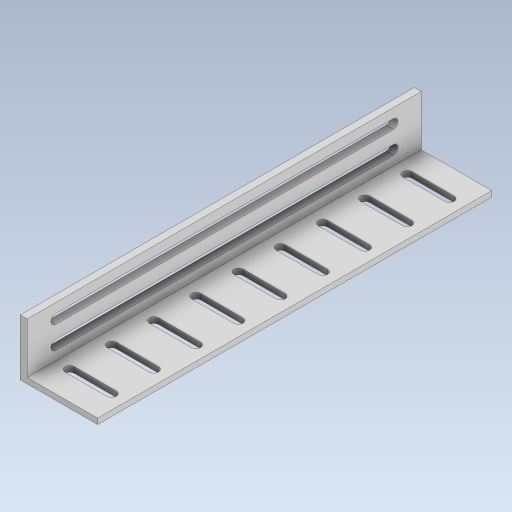
# Autodesk Inventor part: Alas Conveyor
Saved by Autodesk Inventor 2023.5 (Build 275446000, 446)
## iProperties
Created: 2025-10-12
Part Number: Alas Conveyor
Material: Generic
Document SubType Name: Modeling
Designer: Guntur
Density: 1 g/cm^3
Appearance: Default
Author: Guntur
Autodesk Inventor part; units mm, degrees
ref_plane "YZ Plane" through (0, 0, 0) normal (1, 0, 0) x (0, 1, 0)
ref_plane "XZ Plane" through (0, 0, 0) normal (0, 1, 0) x (-1, 0, 0)
ref_plane "XY Plane" through (0, 0, 0) normal (0, 0, 1) x (1, 0, 0)
sketch "Sketch1" plane through (0, 0, 0) normal (0, 1, 0) x (-1, 0, 0)
  line L0 (0, 0) -> (-27.5, 0)
  line L1 (-27.5, 0) -> (-27.5, -140)
  line L2 (-27.5, -140) -> (0, -140)
  line L3 (0, -140) -> (0, 0)
  line L4 (0, 0) -> (-2.5, 0)
  line L5 (-2.5, 0) -> (-2.5, -140)
  line L6 (-2.5, -140) -> (0, -140)
  line L7 (0, -140) -> (0, 0)
  arc A0 (-7.5, -11.65) -> (-7.5, -8.35) centre (-7.5, -10) ccw
  arc A1 (-22.5, -8.35) -> (-22.5, -11.65) centre (-22.5, -10) ccw
  line L8 (-7.5, -11.65) -> (-22.5, -11.65)
  line L9 (-22.5, -8.35) -> (-7.5, -8.35)
  arc A2 (-7.5, -26.65) -> (-7.5, -23.35) centre (-7.5, -25) ccw
  line L10 (-22.5, -23.35) -> (-7.5, -23.35)
  line L11 (-7.5, -26.65) -> (-22.5, -26.65)
  arc A3 (-22.5, -23.35) -> (-22.5, -26.65) centre (-22.5, -25) ccw
  arc A4 (-7.5, -41.65) -> (-7.5, -38.35) centre (-7.5, -40) ccw
  line L12 (-22.5, -38.35) -> (-7.5, -38.35)
  line L13 (-7.5, -41.65) -> (-22.5, -41.65)
  arc A5 (-22.5, -38.35) -> (-22.5, -41.65) centre (-22.5, -40) ccw
  arc A6 (-7.5, -56.65) -> (-7.5, -53.35) centre (-7.5, -55) ccw
  line L14 (-22.5, -53.35) -> (-7.5, -53.35)
  line L15 (-7.5, -56.65) -> (-22.5, -56.65)
  arc A7 (-22.5, -53.35) -> (-22.5, -56.65) centre (-22.5, -55) ccw
  arc A8 (-7.5, -71.65) -> (-7.5, -68.35) centre (-7.5, -70) ccw
  line L16 (-22.5, -68.35) -> (-7.5, -68.35)
  line L17 (-7.5, -71.65) -> (-22.5, -71.65)
  arc A9 (-22.5, -68.35) -> (-22.5, -71.65) centre (-22.5, -70) ccw
  arc A10 (-7.5, -86.65) -> (-7.5, -83.35) centre (-7.5, -85) ccw
  line L18 (-22.5, -83.35) -> (-7.5, -83.35)
  line L19 (-7.5, -86.65) -> (-22.5, -86.65)
  arc A11 (-22.5, -83.35) -> (-22.5, -86.65) centre (-22.5, -85) ccw
  arc A12 (-7.5, -101.65) -> (-7.5, -98.35) centre (-7.5, -100) ccw
  line L20 (-22.5, -98.35) -> (-7.5, -98.35)
  line L21 (-7.5, -101.65) -> (-22.5, -101.65)
  arc A13 (-22.5, -98.35) -> (-22.5, -101.65) centre (-22.5, -100) ccw
  arc A14 (-7.5, -116.65) -> (-7.5, -113.35) centre (-7.5, -115) ccw
  line L22 (-22.5, -113.35) -> (-7.5, -113.35)
  line L23 (-7.5, -116.65) -> (-22.5, -116.65)
  arc A15 (-22.5, -113.35) -> (-22.5, -116.65) centre (-22.5, -115) ccw
  arc A16 (-7.5, -131.65) -> (-7.5, -128.35) centre (-7.5, -130) ccw
  line L24 (-22.5, -128.35) -> (-7.5, -128.35)
  line L25 (-7.5, -131.65) -> (-22.5, -131.65)
  arc A17 (-22.5, -128.35) -> (-22.5, -131.65) centre (-22.5, -130) ccw
  dimension "d0" = 27.5
  dimension "d1" = 140
  dimension "d2" = 2.5
  dimension "d21" = 3.3
  dimension "d22" = 10
  dimension "d23" = 5
  dimension "d24" = 3.3
  dimension "d25" = 5
  dimension "d28" = 15
  constraints: 52 end point, 36 point on circle, 18 centre point, 5 parallel, 3 horizontal, 2 perpendicular, 1 point on line, 1 vertical, 80 other
  measures "d0" distance of L2.end L1.end
  measures "d1" distance of L1.end L0.end
  measures "d2" distance of L6.end L5.end
  measures "d21" diameter of A0
  measures "d22" distance from line of L0 A0.centre
  measures "d23" distance from line of L5 A0.centre
  measures "d24" diameter of A1
  measures "d25" distance from line of L1 A1.centre
  measures "d28" distance of A0.centre A2.centre
extrude "Extrusion1" add sketch "Sketch1" along normal blind 2 contours L5 L2 L1 L0
extrude "Extrusion2" add sketch "Sketch1" along normal blind 20 contours L3 L2 L5 L0
sketch "Sketch2" plane through (2.5, 2, -140) normal (1, 0, 0) x (0, 0, -1)
  circle A0 centre (-130, 5) radius 1.65
  line L0 (0, 0) -> (-140, 0) projected
  circle A1 centre (-130, 13) radius 1.65
  line L1 (-140, 18) -> (0, 18) projected
  line L2 (-140, 0) -> (-140, 18) projected
  line L3 (0, 0) -> (0, 18) projected
  line L4 (-130, 13) -> (-10, 13) construction
  line L5 (-130, 11.35) -> (-10, 11.35)
  line L6 (-10, 14.65) -> (-130, 14.65)
  arc A2 (-130, 14.65) -> (-130, 11.35) centre (-130, 13) ccw
  arc A3 (-10, 11.35) -> (-10, 14.65) centre (-10, 13) ccw
  line L7 (-130, 5) -> (-10, 5) construction
  line L8 (-130, 3.35) -> (-10, 3.35)
  line L9 (-10, 6.65) -> (-130, 6.65)
  arc A4 (-130, 6.65) -> (-130, 3.35) centre (-130, 5) ccw
  arc A5 (-10, 3.35) -> (-10, 6.65) centre (-10, 5) ccw
  point P0 (-140, -2)
  point P1 (-70, 13)
  point P2 (-70, 5)
  point P3 (-130, 6.65)
  point P4 (-130, 3.35)
  point P5 (-130, 14.65)
  point P6 (-130, 11.35)
  dimension "d7" = 3.3
  dimension "d8" = 5
  dimension "d9" = 3.3
  dimension "d10" = 5
  dimension "d11" = 10
  dimension "d12" = 10
  dimension "d15" = 3.3
  dimension "d16" = 3.3
  dimension "d19" = 120
  dimension "d20" = 120
  constraints: 16 end point, 8 point on circle, 8 tangent, 6 centre point, 2 midpoint, 2 parallel, 1 horizontal
  measures "d7" diameter of A0
  measures "d8" distance from line of L0 L7.start
  measures "d9" diameter of A1
  measures "d10" distance from line of L1 L4.start
  measures "d11" distance from line of L2 L4.start
  measures "d12" distance from line of L2 L7.start
  measures "d15" diameter of A3
  measures "d16" diameter of A5
  measures "d19" distance of L6.start L6.end
  measures "d20" distance of L7.start L7.end
extrude "Extrusion3" cut sketch "Sketch2" against normal blind 2.5 contours A0 | A0 L9 A5 L8 | A1 | A1 L6 A3 L5
body "Solid1"
